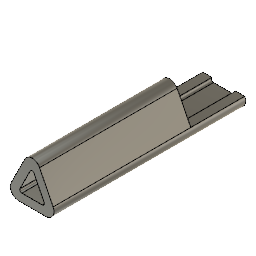
lever_adapter v1 (Autodesk Fusion 360 design; units mm, degrees)
Autodesk Fusion 360 part; units mm, degrees
sketch "Sketch1" plane through (0, 0, 0) normal (0, 1, 0) x (1, 0, 0)
  line L0 (0, 0) -> (6.5, -13)
  line L1 (6.5, -13) -> (13, 0)
  line L2 (13, 0) -> (0, 0)
  line L3 (3.2361, -2) -> (6.5, -8.5279)
  line L4 (6.5, -8.5279) -> (9.7639, -2)
  line L5 (9.7639, -2) -> (3.2361, -2)
  dimension "d1" = 13
  dimension "d2" = 13
  dimension "d3" = 6.5
  dimension "d6" = 2
  dimension "d7" = 2
  dimension "d8" = 2
  constraint coincident L0.start L2.end
  constraint horizontal L2
  constraint parallel L0 L3
  constraint parallel L1 L4
  constraint horizontal L5
  measures "d1" distance of L1.end L0.start
  measures "d2" distance of L0.end L2
  measures "d3" horizontal distance of L0.start L0.end
  measures "d6" distance of L2 L5
  measures "d7" distance of L0 L3
  measures "d8" distance of L1 L4
extrude "Extrude1" add sketch "Sketch1" along normal blind 33
fillet "Fillet1" radius 2 3 edges at (6.5, 16.5, 13) (0, 16.5, 0) (13, 16.5, 0)
fillet "Fillet2" radius 0.5 3 edges at (6.5, 16.5, 8.5279) (3.2361, 16.5, 2) (9.7639, 16.5, 2)
sketch "Sketch2" plane through (0, 33, 0) normal (0, 1, 0) x (-1, 0, 0)
  arc A0 (-11.5528, 2.8944) -> (-9.7639, 0) centre (-9.7639, 2) ccw
  line L0 (-9.7639, 0) -> (-3.2361, 0)
  arc A1 (-3.2361, 0) -> (-1.4472, 2.8944) centre (-3.2361, 2) ccw
  line L1 (-1.4472, 2.8944) -> (-4.7111, 9.4223)
  arc A2 (-4.7111, 9.4223) -> (-8.2889, 9.4223) centre (-6.5, 8.5279) ccw
  line L2 (-8.2889, 9.4223) -> (-11.5528, 2.8944)
  line L3 (-4.0451, 2) -> (-8.9549, 2)
  arc A3 (-9.4021, 2.7236) -> (-8.9549, 2) centre (-8.9549, 2.5) ccw
  line L4 (-9.4021, 2.7236) -> (-6.9472, 7.6334)
  arc A4 (-6.0528, 7.6334) -> (-6.9472, 7.6334) centre (-6.5, 7.4098) ccw
  line L5 (-6.0528, 7.6334) -> (-3.5979, 2.7236)
  arc A5 (-4.0451, 2) -> (-3.5979, 2.7236) centre (-4.0451, 2.5) ccw
  line L6 (-8.9549, 2) -> (-4.0451, 2)
  arc A6 (-3.2361, 0) -> (-1.2361, 2) centre (-3.2361, 2) ccw
  line L7 (-3.2361, 0) -> (-9.7639, 0)
  arc A7 (-11.7639, 2) -> (-9.7639, 0) centre (-9.7639, 2) ccw
  arc A8 (-11.5528, 2.8944) -> (-11.7639, 2) centre (-9.7639, 2) ccw
  arc A9 (-9.3167, 2.8944) -> (-8.9549, 2) centre (-8.9549, 2.5204) ccw
  arc A10 (-4.0451, 2) -> (-3.6833, 2.8944) centre (-4.0451, 2.5204) ccw
  arc A11 (-1.2361, 2) -> (-1.4472, 2.8944) centre (-3.2361, 2) ccw
  line L8 (-11.5528, 2.8944) -> (-9.3167, 2.8944)
  line L9 (-3.6833, 2.8944) -> (-1.4472, 2.8944)
  constraint coincident A0 A7.start
  constraint coincident A1 A6.end
  constraint parallel L3 L6
  constraint coincident L0.end A1.start
  constraint tangent L0 A6
  constraint coincident A0.end L0.start
  constraint tangent L0 A7
  constraint coincident A0.start L2.end
  constraint tangent A7 A8
  constraint coincident L4 A9.start
  constraint coincident L3.end A3.end
  constraint tangent L3 A9
  constraint coincident A1.end L1.start
  constraint coincident L5 A10.end
  constraint coincident A10.end L8
  constraint coincident L3.start A5.start
  constraint tangent L3 A10
  constraint tangent A6 A11
  constraint collinear L8 L9
extrude "Extrude2" add sketch "Sketch2" along normal blind 13 contours A0 L0 A1 L3 L6 A6 L7 A7 A8 A9 A10 A11 L8 L9
